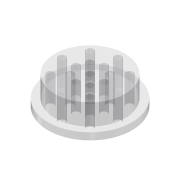
# Autodesk Inventor part: insideFlange
Saved by Autodesk Inventor 2018 (Build 220112000, 112)
## iProperties
Created: 2020-03-26
Part Number: insideFlange
Material: Polycarbonate, Clear
Document SubType Name: Modeling
Designer: Matt
Density: 1.2 g/cm^3
Appearance: Polycarbonate - Clear
Author: Matt
Autodesk Inventor part; units mm, degrees
ref_plane "YZ Plane" through (0, 0, 0) normal (1, 0, 0) x (0, 1, 0)
ref_plane "XZ Plane" through (0, 0, 0) normal (0, 1, 0) x (-1, 0, 0)
ref_plane "XY Plane" through (0, 0, 0) normal (0, 0, 1) x (1, 0, 0)
sketch "Sketch1" plane through (0, 0, 0) normal (0, 1, 0) x (-1, 0, 0)
  circle A0 centre (0, 0) radius 19.05
  circle A1 centre (0, 0) radius 12.7
  dimension "d0" = 38.1
  dimension "d1" = 25.4
  constraints: 2 centre point, 2 coincident
  measures "d0" diameter of A0
  measures "d1" diameter of A1
extrude "Extrusion1" add sketch "Sketch1" along normal blind 3.175
sketch "Sketch2" plane through (0, 3.175, 0) normal (0, 1, 0) x (1, 0, 0)
  circle A0 centre (0, 0) radius 12.7 projected
  circle A1 centre (0, 0) radius 19.05 projected
  circle A2 centre (0, 0) radius 15.875
  dimension "d4" = 31.75
  constraints: 1 centre point, 1 coincident
  measures "d4" diameter of A2
extrude "Extrusion2" add sketch "Sketch2" along normal blind 9.525 contours A2
sketch "Sketch4" plane through (0, 12.7, 0) normal (0, 1, 0) x (1, 0, 0)
  circle A0 centre (0, 0) radius 12.7 projected
  circle A1 centre (0, 0) radius 15.875 projected
extrude "Extrusion4" add sketch "Sketch4" against normal up to surface (12.7 mm away) contours A0
sketch "Sketch5" plane through (0, 0, 0) normal (0, -1, 0) x (1, 0, 0)
  circle A0 centre (-6.35, 0) radius 1.5875 projected
  circle A1 centre (-12.7, 0) radius 1.5875 projected
  circle A2 centre (0, -6.35) radius 1.5875 projected
  circle A3 centre (0, -12.7) radius 1.5875 projected
  circle A4 centre (6.35, 0) radius 1.5875 projected
  circle A5 centre (12.7, 0) radius 1.5875 projected
  circle A6 centre (4.4901, 4.4901) radius 1.5875 projected
  circle A7 centre (8.9803, 8.9803) radius 1.5875 projected
  circle A8 centre (8.9803, -8.9803) radius 1.5875 projected
  circle A9 centre (4.4901, -4.4901) radius 1.5875 projected
  circle A10 centre (-8.9803, -8.9803) radius 1.5875 projected
  circle A11 centre (-4.4901, -4.4901) radius 1.5875 projected
  circle A12 centre (-8.9803, 8.9803) radius 1.5875 projected
  circle A13 centre (-4.4901, 4.4901) radius 1.5875 projected
  circle A14 centre (0, 6.35) radius 1.5875 projected
  circle A15 centre (0, 12.7) radius 1.5875 projected
  circle A16 centre (0, 0) radius 1.5875 projected
  circle A17 centre (0, 0) radius 15.875 projected
extrude "Extrusion5" cut sketch "Sketch5" against normal through all contours A0 | A1 | A2 | A3 | A4 | A5 | A6 | A7 | A8 | A9 | A10 | A11 | A12 | A13 | A14 | A15 | A16
body "Solid1"
